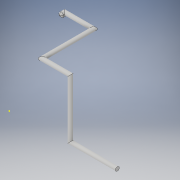
# Autodesk Inventor part: Draht
Saved by Autodesk Inventor 2018 (Build 220112000, 112)
## iProperties
Created: 2018-03-15
Part Number: Draht
Material: Generisch
Document SubType Name: Modeling
Designer: Dominik
Density: 1 g/cm^3
Appearance: Vorgabe
Author: Dominik
Autodesk Inventor part; units mm, degrees
ref_plane "YZ Plane" through (0, 0, 0) normal (1, 0, 0) x (0, 1, 0)
ref_plane "XZ Plane" through (0, 0, 0) normal (0, 1, 0) x (-1, 0, 0)
ref_plane "XY Plane" through (0, 0, 0) normal (0, 0, 1) x (1, 0, 0)
sketch "Skizze1" plane through (0, 0, 0) normal (0, 1, 0) x (-1, 0, 0)
  line L0 (0, 0) -> (70, 0)
  line L1 (70, 0) -> (70, 6)
  line L2 (70, 6) -> (0, 6)
  line L3 (0, 6) -> (0, 0)
  dimension "d0" = 70
  dimension "d1" = 6
  constraints: 8 end point, 2 parallel, 1 horizontal, 1 perpendicular
  measures "d0" distance of L2.end L1.end
  measures "d1" distance of L1.end L0.end
extrude "Extrusion1" add sketch "Skizze1" along normal blind 6
sketch "Skizze2" plane through (0, 0, 0) normal (0, 0, 1) x (1, 0, 0)
  line L0 (0, 0) -> (-70, 0) projected
  line L1 (-70, 0) -> (-76, 0)
  line L2 (-76, 0) -> (-76, 6)
  line L3 (-76, 6) -> (-70, 6)
  line L4 (-70, 6) -> (-70, 0)
  dimension "d4" = 6
  dimension "d5" = 6
  constraints: 8 end point, 2 parallel, 1 horizontal, 1 perpendicular
  measures "d4" distance of L2.end L3.end
  measures "d5" distance of L1.end L2.end
extrude "Extrusion2" add sketch "Skizze2" along normal blind 90
sketch "Skizze3" plane through (0, 0, 90) normal (0, 0, 1) x (1, 0, 0)
  line L0 (-70, 0) -> (0, 0) projected
  line L1 (-70, 0) -> (-120, 0)
  line L2 (-120, 0) -> (-120, 6)
  line L3 (-120, 6) -> (-70, 6)
  line L4 (-70, 6) -> (-70, 0)
  dimension "d8" = 50
  constraints: 8 end point, 2 parallel, 1 horizontal, 1 perpendicular
  measures "d8" distance of L2.end L3.end
extrude "Extrusion3" add sketch "Skizze3" along normal blind 6
sketch "Skizze4" plane through (0, 6, 0) normal (0, 1, 0) x (1, 0, 0)
  line L0 (-120, -90) -> (-76, -90) projected
  line L1 (-70, -96) -> (-120, -96) projected
  line L2 (-120, -90) -> (-114, -90)
  line L3 (-114, -90) -> (-114, -96)
  line L4 (-114, -96) -> (-120, -96)
  line L5 (-120, -96) -> (-120, -90)
  point P0 (0, 0)
  dimension "d11" = 6
  constraints: 8 end point, 2 parallel, 1 horizontal, 1 perpendicular, 1 point on line
  measures "d11" distance of L3.end L4.end
extrude "Extrusion4" add sketch "Skizze4" along normal blind 80
sketch "Skizze5" plane through (-120, 0, 90) normal (-1, 0, 0) x (0, 0, 1)
  line L0 (6, 86) -> (0, 86) projected
  line L1 (0, 0) -> (0, 86) projected
  line L2 (6, 86) -> (0, 86)
  line L3 (0, 86) -> (0, 80)
  line L4 (0, 80) -> (6, 80)
  line L5 (6, 80) -> (6, 86)
  point P0 (-90, 0)
  dimension "d14" = 6
  constraints: 8 end point, 2 parallel, 1 horizontal, 1 perpendicular, 1 point on line
  measures "d14" distance of L3.end L2.end
extrude "Extrusion5" add sketch "Skizze5" along normal blind 45
sketch "Skizze6" plane through (-165, 0, 90) normal (-1, 0, 0) x (0, 0, 1)
  point P0 (-90, 0)
sketch "Skizze7" plane through (-120, 80, 90) normal (0, -1, 0) x (1, 0, 0)
  line L0 (6, 6) -> (-45, 6) projected
  line L1 (6, 0) -> (-45, 0) projected
  line L2 (-45, 6) -> (-39, 6)
  line L3 (-39, 6) -> (-39, 0)
  line L4 (-39, 0) -> (-45, 0)
  line L5 (-45, 0) -> (-45, 6)
  point P0 (120, -90)
  dimension "d17" = 6
  constraints: 8 end point, 2 parallel, 1 horizontal, 1 perpendicular, 1 point on line
  measures "d17" distance of L3.end L4.end
extrude "Extrusion6" add sketch "Skizze7" along normal blind 5
fillet "Rundung1" radius 3 26 edges at (-38, 0, 0) (-38, 6, 0) (-35, 6, 6) (-35, 0, 6) (-70, 0, 51) (-70, 6, 51) (-76, 6, 45) (-76, 0, 45) (-98, 0, 90) (-95, 0, 96) (-92, 6, 96) (-120, 40, 96) (-120, 40, 90) (-114, 46, 90) (-114, 46, 96) (-139.5, 80, 96) (-139.5, 80, 90) (-139.5, 86, 96) (-139.5, 86, 90) (-165, 80.5, 96) (-165, 80.5, 90) (-165, 75, 93) (-159, 75, 93) (-159, 77.5, 96) (-162, 75, 90) (-162, 75, 96)
